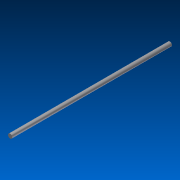
# Autodesk Inventor part: riel
Saved by Autodesk Inventor 2012 (Build 160160000, 160)
## iProperties
Created: 2016-01-04
Part Number: riel
Material: Default
Document SubType Name: Modeling
Designer: Alex Becerra
Mass: 3.7 g
Surface Area: 7.36311 cm^2
Volume: 0.454058 cm^3
Density: 8.14873 g/cm^3
Author: Alex Becerra
Autodesk Inventor part; units mm, degrees
ref_plane "YZ Plane" through (0, 0, 0) normal (1, 0, 0) x (0, 1, 0)
ref_plane "XZ Plane" through (0, 0, 0) normal (0, 1, 0) x (-1, 0, 0)
ref_plane "XY Plane" through (0, 0, 0) normal (0, 0, 1) x (1, 0, 0)
sketch "Sketch1" plane through (0, 0, 0) normal (0, 0, 1) x (1, 0, 0)
  circle A0 centre (0, 0) radius 1.25
  dimension "d0" = 2.5
  dimension "d0" = 2.5
  constraints: 1 centre point, 1 coincident
  measures "d0" diameter of A0
extrude "Extrusion1" add sketch "Sketch1" along normal blind 92.5
body "Solid1"
